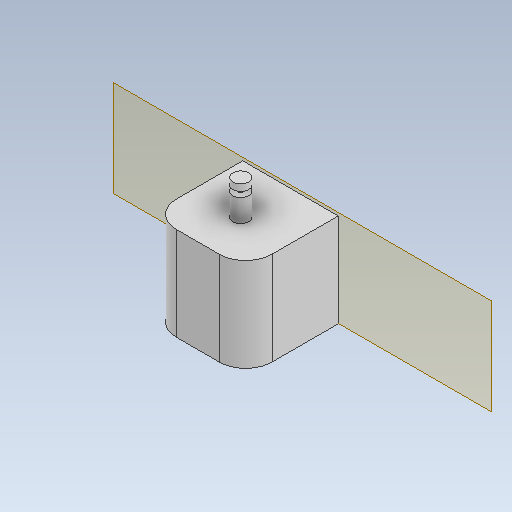
# Autodesk Inventor part: Pieza3
Saved by Autodesk Inventor 2020 (Build 240168000, 168)
## iProperties
Created: 2020-12-08
Part Number: Pieza3
Material: Genérico
Document SubType Name: Modeling
Designer: DanielAlvaradoPelaez
Density: 1 g/cm^3
Appearance: Valor por defecto
Author: DanielAlvaradoPelaez
Autodesk Inventor part; units mm, degrees
ref_plane "YZ Plane" through (0, 0, 0) normal (1, 0, 0) x (0, 1, 0)
ref_plane "XZ Plane" through (0, 0, 0) normal (0, 1, 0) x (-1, 0, 0)
ref_plane "XY Plane" through (0, 0, 0) normal (0, 0, 1) x (1, 0, 0)
ref_plane "Plano de trabajo1" through (-56.2353, 9.9981, -187.965) normal (0, 0, 1) x (1, 0, 0)
sketch "Boceto1" plane through (-56.2353, 9.9981, -187.965) normal (0, 0, 1) x (1, 0, 0)
  line L0 (-114.1422, 169.9991) -> (-475.1878, 169.9991)
  line L1 (-475.1878, 169.9991) -> (-475.1878, -182.9514)
  line L2 (-475.1878, -182.9514) -> (-114.1422, -182.9514)
  line L3 (-114.1422, -182.9514) -> (-114.1422, 169.9991)
  point P0 (56.2353, -9.9981)
  constraints: 8 end point, 2 parallel, 1 horizontal, 1 perpendicular
extrude "Extrusión1" add sketch "Boceto1" along normal blind 350
fillet "Empalme1" radius 100 2 edges at (-531.4231, 3.522, 162.035) (-170.3775, 3.522, 162.035)
sketch "Boceto2" plane through (-531.4231, 179.9972, -187.965) normal (0, 1, 0) x (1, 0, 0)
  circle A0 centre (180.5228, -187.965) radius 30
  point P0 (531.4231, -187.965)
  dimension "d3" = 60
  constraints: 1 centre point
  measures "d3" diameter of A0
extrude "Extrusión2" add sketch "Boceto2" along normal blind 85
sketch "Boceto5" plane through (-350.9003, 264.9972, 0) normal (0, 1, 0) x (1, 0, 0)
  circle A0 centre (0, 0) radius 7.5
  point P0 (350.9003, 0)
  dimension "d18" = 15
  constraints: 1 centre point
  measures "d18" diameter of A0
extrude "Extrusión5" add sketch "Boceto5" along normal blind 20
sketch "Boceto6" plane through (-350.9003, 284.9972, 0) normal (0, 1, 0) x (1, 0, 0)
  circle A0 centre (0, 0) radius 7.5 projected
  circle A1 centre (0, 0) radius 30
  point P0 (350.9003, 0)
  dimension "d21" = 60
  constraints: 1 centre point, 1 coincident
  measures "d21" diameter of A1
extrude "Extrusión6" add sketch "Boceto6" along normal blind 25 contours A0 | A1
